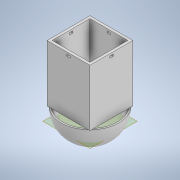
# Autodesk Inventor part: box-v1
Saved by Autodesk Inventor 2022 (Build 260153000, 153)
## iProperties
Created: 2021-07-14
Part Number: box-v1
Material: Generic
Document SubType Name: Modeling
Designer: dncob
Density: 1 g/cm^3
Appearance: Default
Author: dncob
Autodesk Inventor part; units mm, degrees
ref_plane "YZ Plane" through (0, 0, 0) normal (1, 0, 0) x (0, 1, 0)
ref_plane "XZ Plane" through (0, 0, 0) normal (0, 1, 0) x (-1, 0, 0)
ref_plane "XY Plane" through (0, 0, 0) normal (0, 0, 1) x (1, 0, 0)
sketch "Sketch1" plane through (0, 0, 0) normal (0, 1, 0) x (-1, 0, 0)
  line L0 (-30, 30) -> (30, 30)
  line L1 (30, 30) -> (30, -30)
  line L2 (30, -30) -> (-30, -30)
  line L3 (-30, -30) -> (-30, 30)
  line L4 (-30, 30) -> (30, -30) construction
  line L5 (30, 30) -> (-30, -30) construction
  line L6 (-34, 34) -> (34, 34)
  line L7 (34, 34) -> (34, -34)
  line L8 (34, -34) -> (-34, -34)
  line L9 (-34, -34) -> (-34, 34)
  line L10 (-34, 34) -> (34, -34) construction
  line L11 (34, 34) -> (-34, -34) construction
  point P0 (0, 0)
  dimension "d0" = 60
  dimension "d1" = 4
  dimension "d2" = 4
  constraints: 24 end point, 4 midpoint, 4 parallel, 3 perpendicular, 2 horizontal
  measures "d0" distance of L0.end L1.end
  measures "d1" distance between parallel lines of L1 L7
  measures "d2" distance between parallel lines of L0 L6
extrude "Extrusion1" add sketch "Sketch1" along normal blind 90
sketch "Sketch2" plane through (34, 0, 34) normal (1, 0, 0) x (0, 0, -1)
  line L0 (31.5, 87) -> (36.5, 87)
  line L1 (36.5, 87) -> (36.5, 84)
  line L2 (36.5, 84) -> (31.5, 84)
  line L3 (31.5, 84) -> (31.5, 87)
  line L4 (31.5, 87) -> (36.5, 84) construction
  line L5 (36.5, 87) -> (31.5, 84) construction
  line L6 (0, 90) -> (68, 90) projected
  point P0 (34, 0)
  point P1 (34, 85.5)
  dimension "d5" = 3
  dimension "d6" = 3
  dimension "d7" = 5
  constraints: 12 end point, 2 midpoint, 2 parallel, 1 horizontal, 1 perpendicular, 1 vertical alignment
  measures "d5" distance between parallel lines of L0 L6
  measures "d6" distance of L0.end L1.end
  measures "d7" distance of L1.end L2.end
extrude "Extrusion2" cut sketch "Sketch2" against normal up to surface (4 mm away)
pattern_circular "Circular Pattern1" count 4 over 360 about axis through (0, -10, 0) along (0, 1, 0) of "Extrusion2"
sketch "Sketch3" plane through (0, 0, 0) normal (0, -1, 0) x (1, 0, 0)
  arc A0 (-43.6, 0) -> (43.6, 0) centre (0, 0) ccw
  arc A1 (-46.1, 0) -> (46.1, 0) centre (0, 0) ccw
  line L0 (43.6, 0) -> (46.1, 0)
  line L1 (-46.1, 0) -> (-43.6, 0)
  line L2 (0, 0) -> (7.0498, 0) construction
  dimension "d14" = 2.5
  dimension "d17" = 43.6
  constraints: 6 end point, 4 point on circle, 3 horizontal, 2 centre point, 2 coincident, 2 collinear
  measures "d14" radial gap between concentric circles of A0 A1
  measures "d17" radius of A0
revolve "Revolution1" add sketch "Sketch3" angle 180 about axis through (0, 0, 0) along (-1, 0, 0)
ref_plane "Work Plane1" through (0, -21, 0) normal (0, -1, 0) x (1, 0, 0)
body "Solid1"
